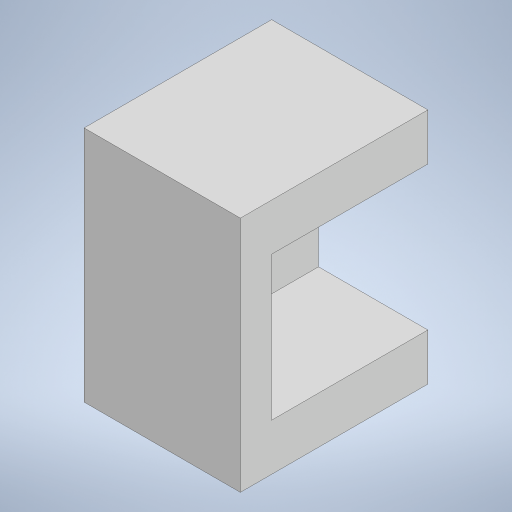
# Autodesk Inventor part: ограничитель
Saved by Autodesk Inventor 2023.1 (Build 271208000, 208)
## iProperties
Created: 2025-01-24
Part Number: ограничитель
Material: Типовые
Document SubType Name: Modeling
Designer: DELL
Density: 1 g/cm^3
Appearance: По умолчанию
Author: DELL
Autodesk Inventor part; units mm, degrees
ref_plane "YZ Plane" through (0, 0, 0) normal (1, 0, 0) x (0, 1, 0)
ref_plane "XZ Plane" through (0, 0, 0) normal (0, 1, 0) x (-1, 0, 0)
ref_plane "XY Plane" through (0, 0, 0) normal (0, 0, 1) x (1, 0, 0)
sketch "Эскиз1" plane through (0, 0, 0) normal (0, 0, 1) x (1, 0, 0)
  line L0 (4.6286, 7.4989) -> (-5.3714, 7.4989)
  line L1 (-5.3714, 7.4989) -> (-5.3714, -7.7011)
  line L2 (-5.3714, -7.7011) -> (4.6286, -7.7011)
  line L3 (4.6286, -7.7011) -> (4.6286, -4.7011)
  line L4 (4.6286, -4.7011) -> (-2.3714, -4.7011)
  line L5 (-2.3714, 4.4989) -> (4.6286, 4.4989)
  line L6 (4.6286, 4.4989) -> (4.6286, 7.4989)
  line L7 (-2.3714, 4.4989) -> (-2.3714, -4.7011)
  point P0 (0, 0)
  dimension "d1" = 9.2
  dimension "d2" = 3
  dimension "d3" = 3
  dimension "d4" = 3
  dimension "d7" = 10
  constraints: 17 end point, 5 perpendicular, 2 parallel, 1 horizontal, 1 vertical
  measures "d1" distance of L5.start L4.end
  measures "d2" distance of L5.end L0.start
  measures "d3" distance of L2.end L3.end
  measures "d4" distance between parallel lines of L1 L7
  measures "d7" distance of L1.end L2.end
extrude "Выдавливание1" add sketch "Эскиз1" along normal blind 10
sketch "Эскиз3" plane through (0, 0, 10) normal (0, 0, 1) x (1, 0, 0)
  line L0 (4.6286, 7.4989) -> (-5.3714, 7.4989) projected
  line L1 (4.6286, -7.7011) -> (4.6286, -4.7011) projected
  line L2 (-5.3714, 7.4989) -> (4.6286, 7.4989)
  line L3 (4.6286, 7.4989) -> (4.6286, -7.7011)
  line L4 (4.6286, -7.7011) -> (-5.3714, -7.7011)
  line L5 (-5.3714, -7.7011) -> (-5.3714, 7.4989)
  point P0 (0, 0)
  point P1 (4.6286, 7.4989)
  constraints: 8 end point, 2 parallel, 1 horizontal, 1 perpendicular
extrude "Выдавливание3" add sketch "Эскиз3" along normal blind 2
